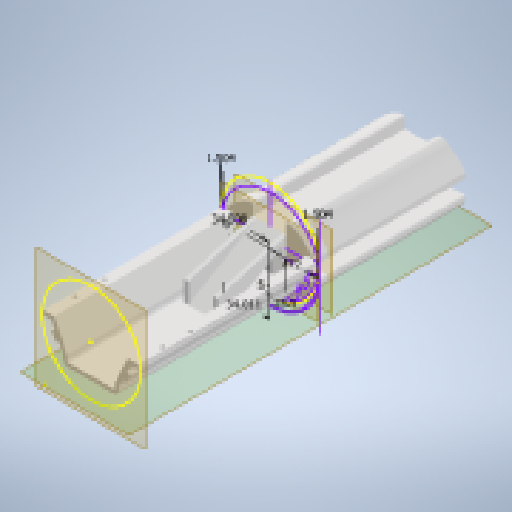
# Autodesk Inventor part: MiddleAdapter_0.5mmOffset
Saved by Autodesk Inventor 2023 (Build 270158030, 158C)
## iProperties
Created: 2022-07-21
Part Number: MiddleAdapter_0.5mmOffset
Material: Generic
Document SubType Name: Modeling
Designer: sqa4002
Density: 1 g/cm^3
Appearance: Default
Author: sqa4002
Autodesk Inventor part; units mm, degrees
ref_plane "YZ Plane" through (0, 0, 0) normal (1, 0, 0) x (0, 1, 0)
ref_plane "XZ Plane" through (0, 0, 0) normal (0, 1, 0) x (-1, 0, 0)
ref_plane "XY Plane" through (0, 0, 0) normal (0, 0, 1) x (1, 0, 0)
sketch "Sketch1" plane through (0, 0, 0) normal (0, 0, 1) x (1, 0, 0)
  arc A0 (19, 57.068098) -> (5, 45.931677) centre (29.5, 29.5) ccw
  arc A1 (63, 45.931677) -> (49, 57.068098) centre (38.5, 29.5) ccw
  line L0 (49, 57.068098) -> (49, 49)
  line L1 (49, 49) -> (19, 49)
  line L2 (19, 49) -> (19, 57.068098)
  line L3 (51, 39.215827) -> (51, 45.931677)
  line L4 (51, 45.931677) -> (63, 45.931677)
  line L5 (5, 45.931677) -> (17, 45.931677)
  line L6 (17, 29) -> (5, 29)
  line L7 (63, 29) -> (51, 29)
  line L8 (51, 29) -> (51, 35.71585)
  line L9 (51, 35.71585) -> (41, 35.71585)
  line L10 (41, 35.71585) -> (41, 39.215827)
  line L11 (41, 39.215827) -> (51, 39.215827)
  line L12 (17, 45.931677) -> (17, 39.215827)
  line L13 (17, 39.215827) -> (27, 39.215827)
  line L14 (27, 39.215827) -> (27, 35.715827)
  line L15 (27, 35.715827) -> (17, 35.715827)
  line L16 (17, 35.715827) -> (17, 29)
  arc A2 (5, 29) -> (63, 29) centre (34, 49.533333) ccw
  point P0 (0, 0)
  point P1 (17, 44.965827)
  point P2 (17, 35.465827)
  point P3 (17, 29.465827)
  point P4 (51, 29.465827)
  point P5 (51, 35.465827)
  point P6 (29.5, 29.5)
  point P7 (38.5, 29.5)
sketch "Sketch7" plane through (0, 0, 0) normal (0, 0, 1) x (1, 0, 0)
  arc A0 (19, 57.068098) -> (5, 45.931677) centre (29.5, 29.5) ccw
  arc A1 (63, 45.931677) -> (49, 57.068098) centre (38.5, 29.5) ccw
  line L0 (49, 57.068098) -> (49, 49)
  line L1 (49, 49) -> (19, 49)
  line L2 (19, 49) -> (19, 57.068098)
  arc A2 (5, 29) -> (63, 29) centre (34, 49.533333) ccw
  line L3 (63, 29) -> (51, 29)
  line L4 (51, 29) -> (51, 35.71585)
  line L5 (51, 29) -> (51, 45.931677)
  line L6 (51, 45.931677) -> (63, 45.931677)
  line L7 (5, 45.931677) -> (17, 45.931677)
  line L8 (17, 45.931677) -> (17, 29)
  line L9 (17, 35.715827) -> (17, 29)
  line L10 (17, 29) -> (5, 29)
  point P0 (0, 0)
  point P1 (0, 0)
  point P2 (38.5, 29.5)
  point P3 (51, 44.965827)
  point P4 (17, 44.965827)
  point P5 (17, 35.465827)
  point P6 (17, 29.465827)
  point P7 (51, 29.465827)
  point P8 (51, 35.465827)
  constraints: 22 end point, 6 point on circle, 3 centre point
sketch "Sketch8" plane through (0, 0, 0) normal (0, 0, 1) x (1, 0, 0)
  line L0 (16.4, 45.331677) -> (16.4, 29.6)
  line L1 (16.4, 29.6) -> (3.862316, 29.6)
  arc A0 (3.862316, 29.6) -> (64.137684, 29.6) centre (34, 49.533333) ccw
  line L2 (64.137684, 29.6) -> (51.6, 29.6)
  line L3 (51.6, 29.6) -> (51.6, 45.331677)
  line L4 (51.6, 45.331677) -> (64.100156, 45.331677)
  arc A1 (64.100156, 45.331677) -> (48.4, 57.925341) centre (38.5, 29.5) ccw
  line L5 (48.4, 57.925341) -> (48.4, 49.6)
  line L6 (48.4, 49.6) -> (19.6, 49.6)
  line L7 (19.6, 49.6) -> (19.6, 57.925341)
  arc A2 (19.6, 57.925341) -> (3.899844, 45.331677) centre (29.5, 29.5) ccw
  line L8 (3.899844, 45.331677) -> (16.4, 45.331677)
  line L9 (13.9, 42.831677) -> (13.9, 32.1)
  line L10 (13.9, 32.1) -> (1.670629, 32.1)
  line L11 (1.670629, 32.1) -> (1.670629, 28.382773)
  arc A3 (1.670629, 28.382773) -> (66.329371, 28.382773) centre (34, 49.533333) ccw
  line L12 (66.329371, 28.382773) -> (66.329371, 32.1)
  line L13 (66.329371, 32.1) -> (54.1, 32.1)
  line L14 (54.1, 32.1) -> (54.1, 42.831677)
  line L15 (54.1, 42.831677) -> (66.314291, 42.831677)
  line L16 (66.314291, 42.831677) -> (66.314291, 46.503682)
  arc A4 (66.314291, 46.503682) -> (49.244541, 60.27848) centre (38.5, 29.5) ccw
  line L17 (49.244541, 60.27848) -> (45.9, 60.27848)
  line L18 (45.9, 60.27848) -> (45.9, 52.1)
  line L19 (45.9, 52.1) -> (22.1, 52.1)
  line L20 (22.1, 52.1) -> (22.1, 60.27848)
  line L21 (22.1, 60.27848) -> (18.755459, 60.27848)
  arc A5 (18.755459, 60.27848) -> (1.685709, 46.503682) centre (29.5, 29.5) ccw
  line L22 (1.685709, 46.503682) -> (1.685709, 42.831677)
  line L23 (1.685709, 42.831677) -> (13.9, 42.831677)
  point P0 (0, 0)
  point P1 (38.5, 29.5)
  constraints: 48 end point, 12 point on circle, 6 centre point, 6 perpendicular
extrude "Extrusion3" add sketch "Sketch8" along normal blind 100
ref_plane "Work Plane3" through (0, 0, 100) normal (0, 0, 1) x (1, 0, 0)
sketch "Sketch10" plane through (0, 0, 100) normal (0, 0, 1) x (1, 0, 0)
  line L0 (2.035709, 46.404887) -> (2.035709, 43.181677)
  line L1 (2.035709, 43.181677) -> (14.25, 43.181677)
  line L2 (14.25, 43.181677) -> (14.25, 31.75)
  line L3 (14.25, 31.75) -> (2.020629, 31.75)
  line L4 (2.020629, 31.75) -> (2.020629, 28.48735)
  arc A0 (2.020629, 28.48735) -> (65.979371, 28.48735) centre (34, 49.533333) ccw
  line L5 (65.979371, 28.48735) -> (65.979371, 31.75)
  line L6 (65.979371, 31.75) -> (53.75, 31.75)
  line L7 (53.75, 31.75) -> (53.75, 43.181677)
  line L8 (53.75, 43.181677) -> (65.964291, 43.181677)
  line L9 (65.964291, 43.181677) -> (65.964291, 46.404887)
  arc A1 (65.964291, 46.404887) -> (49.185041, 59.92848) centre (38.5, 29.5) ccw
  line L10 (49.185041, 59.92848) -> (46.25, 59.92848)
  line L11 (46.25, 59.92848) -> (46.25, 51.75)
  line L12 (46.25, 51.75) -> (21.75, 51.75)
  line L13 (21.75, 51.75) -> (21.75, 59.92848)
  line L14 (21.75, 59.92848) -> (18.814959, 59.92848)
  arc A2 (18.814959, 59.92848) -> (2.035709, 46.404887) centre (29.5, 29.5) ccw
  line L15 (4.520629, 29.25) -> (16.75, 29.25)
  line L16 (16.75, 29.25) -> (16.75, 45.681677)
  line L17 (16.75, 45.681677) -> (4.535709, 45.681677)
  arc A3 (19.25, 57.42848) -> (4.535709, 45.681677) centre (29.5, 29.5) ccw
  line L18 (19.25, 57.42848) -> (19.25, 49.25)
  line L19 (19.25, 49.25) -> (48.75, 49.25)
  line L20 (48.75, 49.25) -> (48.75, 57.42848)
  arc A4 (63.464291, 45.681677) -> (48.75, 57.42848) centre (38.5, 29.5) ccw
  line L21 (63.464291, 45.681677) -> (51.25, 45.681677)
  line L22 (51.25, 45.681677) -> (51.25, 29.25)
  line L23 (51.25, 29.25) -> (63.479371, 29.25)
  arc A5 (4.520629, 29.25) -> (63.479371, 29.25) centre (34, 49.533333) ccw
  line L24 (13.9, 32.1) -> (1.670629, 32.1)
  line L25 (1.670629, 32.1) -> (1.670629, 28.382773)
  arc A6 (1.670629, 28.382773) -> (66.329371, 28.382773) centre (34, 49.533333) ccw
  line L26 (66.329371, 28.382773) -> (66.329371, 32.1)
  line L27 (66.329371, 32.1) -> (54.1, 32.1)
  line L28 (54.1, 32.1) -> (54.1, 42.831677)
  line L29 (54.1, 42.831677) -> (66.314291, 42.831677)
  line L30 (66.314291, 42.831677) -> (66.314291, 46.503682)
  arc A7 (66.314291, 46.503682) -> (49.244541, 60.27848) centre (38.5, 29.5) ccw
  line L31 (49.244541, 60.27848) -> (45.9, 60.27848)
  line L32 (45.9, 60.27848) -> (45.9, 52.1)
  line L33 (45.9, 52.1) -> (22.1, 52.1)
  line L34 (22.1, 52.1) -> (22.1, 60.27848)
  line L35 (22.1, 60.27848) -> (18.755459, 60.27848)
  arc A8 (18.755459, 60.27848) -> (1.685709, 46.503682) centre (29.5, 29.5) ccw
  line L36 (1.685709, 46.503682) -> (1.685709, 42.831677)
  line L37 (1.685709, 42.831677) -> (13.9, 42.831677)
  line L38 (13.9, 42.831677) -> (13.9, 32.1)
  line L39 (16.4, 45.331677) -> (3.899844, 45.331677)
  arc A9 (19.6, 57.925341) -> (3.899844, 45.331677) centre (29.5, 29.5) ccw
  line L40 (19.6, 57.925341) -> (19.6, 49.6)
  line L41 (19.6, 49.6) -> (48.4, 49.6)
  line L42 (48.4, 49.6) -> (48.4, 57.925341)
  arc A10 (64.100156, 45.331677) -> (48.4, 57.925341) centre (38.5, 29.5) ccw
  line L43 (64.100156, 45.331677) -> (51.6, 45.331677)
  line L44 (51.6, 45.331677) -> (51.6, 29.6)
  line L45 (51.6, 29.6) -> (64.137684, 29.6)
  arc A11 (3.862316, 29.6) -> (64.137684, 29.6) centre (34, 49.533333) ccw
  line L46 (3.862316, 29.6) -> (16.4, 29.6)
  line L47 (16.4, 29.6) -> (16.4, 45.331677)
  point P0 (0, 0)
extrude "Extrusion4" add sketch "Sketch10" along normal blind 10 contours A2 L14 L13 L12 L11 L10 A1 L9 L8 L7 L6 L5 A0 L4 L3 L2 L1 L0 | L15 L16 L17 A3 L18 L19 L20 A4 L21 L22 L23 A5 | L38 L37 L36 A8 L35 L34 L33 L32 L31 A7 L30 L29 L28 L27 L26 A6 L25 L24 | L39 A9 L40 L41 L42 A10 L43 L44 L45 A11 L46 L47
sketch "Sketch11" plane through (0, 0, 110) normal (0, 0, 1) x (1, 0, 0)
  line L0 (5.317303, 37.465838) -> (7.794293, 32.202234)
  line L1 (7.794293, 32.202234) -> (5.351283, 31.052582)
  line L2 (5.351283, 31.052582) -> (8.331862, 24.718851)
  line L3 (8.331862, 24.718851) -> (10.774872, 25.868503)
  line L4 (10.774872, 25.868503) -> (13.5, 20.077607)
  line L5 (13.5, 20.077607) -> (13.5, 17.965838)
  arc A0 (13.5, 17.965838) -> (18, 13.465838) centre (18, 17.965838) ccw
  line L6 (18, 13.465838) -> (50, 13.465838)
  arc A1 (50, 13.465838) -> (54.5, 17.965838) centre (50, 17.965838) ccw
  line L7 (54.5, 17.965838) -> (54.5, 20.077607)
  line L8 (54.5, 20.077607) -> (57.225128, 25.868503)
  line L9 (57.225128, 25.868503) -> (59.668138, 24.718851)
  line L10 (59.668138, 24.718851) -> (62.648717, 31.052582)
  line L11 (62.648717, 31.052582) -> (60.205707, 32.202234)
  line L12 (60.205707, 32.202234) -> (62.682697, 37.465838)
  line L13 (62.682697, 37.465838) -> (68.496377, 37.465838)
  arc A2 (-0.496377, 37.465838) -> (68.496377, 37.465838) centre (34, 36.965838) ccw
  line L14 (-0.496377, 37.465838) -> (5.317303, 37.465838)
  circle A3 centre (34, 8.465838) radius 2.75
  circle A4 centre (34.011144, 37.465838) radius 36
  line L15 (34.011144, 1.465838) -> (34.011144, 73.465838)
  line L16 (70.011144, 37.465838) -> (-1.988856, 37.465838)
  line L17 (69.999977, 73.499564) -> (69.999977, 1.499564)
  line L18 (-1.999977, 1.499564) -> (-1.999977, 73.499564)
  point P0 (0, 0)
  point P1 (-1.48044, 45.569992)
  point P2 (34, 13.465838)
  point P3 (69.48044, 45.569992)
  point P4 (-0.443994, 38.930856)
  point P5 (68.443994, 38.930856)
  point P6 (0.816224, 46.40443)
  point P7 (67.183776, 46.40443)
  point P8 (0, 0)
  dimension "d27" = 5
  dimension "d28" = 28.5
  dimension "d31" = 72
  dimension "d35" = 1.5036
  dimension "d36" = 1.5036
  dimension "d37" = 34.50752
  dimension "d38" = 0
  dimension "d39" = 34.01114
  constraints: 38 end point, 14 point on circle, 5 centre point, 2 perpendicular, 2 point on line, 2 vertical, 1 midpoint
  measures "d27" distance of point (34, 13.466) A3.centre
  measures "d28" distance of A2.centre A3.centre
  measures "d31" diameter of A4
  measures "d35" distance from line of L18 L14.start
  measures "d36" distance from line of L17 L13.end
  measures "d37" distance of A4.centre L14.start
  measures "d38" distance between parallel lines of L16 L14
  measures "d39" horizontal distance of point (0, 0) A4.centre
sketch "Sketch12" plane through (0, 0, 110) normal (0, 0, 1) x (1, 0, 0)
  circle A0 centre (34, 43.5) radius 36
  line L0 (34, 79.5) -> (34, 7.5)
  line L1 (70, 43.5) -> (-2, 43.5)
  arc A1 (-0.496377, 43.5) -> (68.496377, 43.5) centre (34, 43) ccw
  line L2 (5.317303, 43.5) -> (7.794293, 38.236396)
  line L3 (7.794293, 38.236396) -> (5.351283, 37.086744)
  line L4 (5.351283, 37.086744) -> (8.331862, 30.753013)
  line L5 (8.331862, 30.753013) -> (10.774872, 31.902665)
  line L6 (10.774872, 31.902665) -> (13.5, 26.111768)
  line L7 (13.5, 26.111768) -> (13.5, 24)
  arc A2 (13.5, 24) -> (18, 19.5) centre (18, 24) ccw
  line L8 (18, 19.5) -> (50, 19.5)
  arc A3 (50, 19.5) -> (54.5, 24) centre (50, 24) ccw
  line L9 (54.5, 24) -> (54.5, 26.111768)
  line L10 (54.5, 26.111768) -> (57.225128, 31.902665)
  line L11 (57.225128, 31.902665) -> (59.668138, 30.753013)
  line L12 (59.668138, 30.753013) -> (62.648717, 37.086744)
  line L13 (62.648717, 37.086744) -> (60.205707, 38.236396)
  line L14 (60.205707, 38.236396) -> (62.682697, 43.5)
  line L15 (62.682697, 43.5) -> (68.496377, 43.5)
  circle A4 centre (34, 14.5) radius 2.75
  line L16 (5.317303, 43.5) -> (-0.496377, 43.5)
  point P0 (0, 0)
  point P1 (-0.250325, 38.856906)
  point P2 (68.250325, 38.856906)
  point P3 (-0.329941, 46.421278)
  point P4 (68.329941, 46.421278)
  point P5 (0.881853, 46.584282)
  point P6 (34, 19.5)
  point P7 (67.118147, 46.584282)
  dimension "d42" = 5
  dimension "d43" = 28.5
  dimension "d44" = 0
  constraints: 34 end point, 14 point on circle, 4 centre point, 2 point on line, 1 horizontal, 1 midpoint, 1 vertical
  measures "d42" distance of point (34, 19.5) A4.centre
  measures "d43" distance of A1.centre A4.centre
  measures "d44" distance between parallel lines of L1 L16
ref_plane "Work Plane4" through (0, 0, 110) normal (0, 0, 1) x (1, 0, 0)
sketch "Sketch13" plane through (0, 0, 110) normal (0, 0, 1) x (1, 0, 0)
  circle A0 centre (34, 43.5) radius 36
  line L0 (34, 79.5) -> (34, 7.5)
  line L1 (70, 43.5) -> (-2, 43.5)
  line L2 (5.467102, 43.181677) -> (14.25, 43.181677)
  line L3 (5.317303, 43.5) -> (7.794293, 38.236396)
  arc A1 (-0.496377, 43.5) -> (68.496377, 43.5) centre (34, 43) ccw
  line L4 (7.794293, 38.236396) -> (5.351283, 37.086744)
  line L5 (5.351283, 37.086744) -> (8.331862, 30.753013)
  line L6 (8.331862, 30.753013) -> (10.774872, 31.902665)
  line L7 (10.774872, 31.902665) -> (13.5, 26.111768)
  line L8 (13.5, 26.111768) -> (13.5, 24)
  arc A2 (13.5, 24) -> (18, 19.5) centre (18, 24) ccw
  line L9 (18, 19.5) -> (50, 19.5)
  circle A3 centre (34, 14.5) radius 2.75
  arc A4 (50, 19.5) -> (54.5, 24) centre (50, 24) ccw
  line L10 (54.5, 24) -> (54.5, 26.111768)
  line L11 (54.5, 26.111768) -> (57.225128, 31.902665)
  line L12 (57.225128, 31.902665) -> (59.668138, 30.753013)
  line L13 (59.668138, 30.753013) -> (62.648717, 37.086744)
  line L14 (62.648717, 37.086744) -> (60.205707, 38.236396)
  line L15 (60.205707, 38.236396) -> (62.682697, 43.5)
  line L16 (62.682697, 43.5) -> (68.496377, 43.5)
  line L17 (5.317303, 43.5) -> (-0.496377, 43.5)
  line L18 (5.467102, 43.181677) -> (14.25, 43.181677)
  line L19 (14.25, 43.181677) -> (14.25, 31.75)
  line L20 (14.25, 31.75) -> (2.020629, 31.75)
  line L21 (2.020629, 31.75) -> (2.020629, 28.48735)
  arc A5 (2.020629, 28.48735) -> (65.979371, 28.48735) centre (34, 49.533333) ccw
  line L22 (65.979371, 28.48735) -> (65.979371, 31.75)
  line L23 (65.979371, 31.75) -> (53.75, 31.75)
  line L24 (53.75, 31.75) -> (53.75, 43.181677)
  line L25 (53.75, 43.181677) -> (62.532898, 43.181677)
  line L26 (49.185041, 59.92848) -> (46.25, 59.92848)
  line L27 (46.25, 59.92848) -> (46.25, 51.75)
  line L28 (46.25, 51.75) -> (21.75, 51.75)
  line L29 (21.75, 51.75) -> (21.75, 59.92848)
  line L30 (21.75, 59.92848) -> (18.814959, 59.92848)
  line L31 (12.211937, 35.894512) -> (7.181457, 46.584282)
  line L32 (60.77832, 46.584282) -> (55.788063, 35.894512)
  line L33 (55.788063, 35.894512) -> (51.5, 26.782379)
  line L34 (51.5, 26.782379) -> (51.5, 24)
  arc A6 (50, 22.5) -> (51.5, 24) centre (50, 24) ccw
  line L35 (50, 22.5) -> (18, 22.5)
  arc A7 (16.5, 24) -> (18, 22.5) centre (18, 24) ccw
  line L36 (16.5, 24) -> (16.5, 26.782379)
  line L37 (16.5, 26.782379) -> (12.211937, 35.894512)
  arc A8 (67.118147, 46.584282) -> (49.185041, 59.92848) centre (44.1845, 34.486172) ccw
  arc A9 (18.814959, 59.92848) -> (0.881853, 46.584282) centre (23.8155, 34.486172) ccw
  line L38 (7.181457, 46.584282) -> (0.881853, 46.584282)
  line L39 (60.77832, 46.584282) -> (67.118147, 46.584282)
  line L40 (-0.496377, 43.5) -> (-0.496377, 46.584282)
  line L41 (-0.496377, 46.584282) -> (0.881853, 46.584282)
  line L42 (68.496377, 43.5) -> (68.496377, 46.584282)
  line L43 (68.496377, 46.584282) -> (67.118147, 46.584282)
  point P0 (0, 0)
  point P1 (0, 0)
  point P2 (-0.250325, 38.856906)
  point P3 (68.250325, 38.856906)
  point P4 (-0.329941, 46.421278)
  point P5 (68.329941, 46.421278)
  point P6 (34, 19.5)
  point P7 (-0.496377, 43.5)
  point P8 (68.496377, 43.5)
  dimension "d46" = 5
  dimension "d47" = 28.5
  dimension "d48" = 0
  constraints: 88 end point, 24 point on circle, 10 centre point, 4 point on line, 2 collinear, 2 perpendicular, 2 vertical, 1 horizontal, 1 midpoint, 1 parallel, 6 other
  measures "d46" distance of point (34, 19.5) A3.centre
  measures "d47" distance of A1.centre A3.centre
  measures "d48" distance between parallel lines of L1 L17
extrude "Extrusion5" add sketch "Sketch13" along normal blind 130 contours L1 L32 L39 L43 L42 | L15 L25 L32 L1 | L40 L41 L38 L31 L1 | L15 L14 L13 L23 L12 L11 L33 L32 L25 | L1 L31 L2 L3 | L35 A6 L34 L33 L23 L11 L10 A4 L9 L0 | L0 L9 A2 L8 L7 L20 L37 L36 A7 L35 | L13 L12 L23 | L2 L31 L37 L20 L7 L6 L5 L4 L3 | L20 L6 L5
sketch "Sketch14" plane through (18, 22.5, 110) normal (0, 1, 0) x (1, 0, 0)
  line L0 (28.25, 0) -> (3.75, 0) projected
  line L1 (3.75, 0) -> (28.25, 0)
  line L2 (0, 0) -> (32, 0) projected
  line L3 (28.25, 0) -> (28.25, -50)
  line L4 (32, 0) -> (32, -130) projected
  line L5 (32, -130) -> (0, -130) projected
  line L6 (3.75, 0) -> (3.75, -50)
  line L7 (32, 0) -> (0, 0) projected
  line L8 (25.25, -50) -> (25.25, 0)
  line L9 (6.75, 0) -> (6.75, -50)
  line L10 (28.25, -50) -> (25.25, -50)
  line L11 (6.75, -50) -> (3.75, -50)
  point P0 (-18, 110)
  dimension "d62" = 3
  dimension "d121" = 50
  constraints: 14 end point, 6 point on line, 2 perpendicular, 1 collinear, 1 parallel
  measures "d62" distance between parallel lines of L6 L9
  measures "d121" distance between parallel lines of L0 L10
ref_plane "Work Plane5" through (24.75, 22.5, 110) normal (0, 1, 0) x (1, 0, 0)
sketch "Sketch15" plane through (24.75, 22.5, 110) normal (0, 1, 0) x (1, 0, 0)
  line L0 (0, 0) -> (18.5, 0) projected
  line L1 (18.5, 0) -> (18.5, -130) projected
  line L2 (0, 0) -> (18.5, 0)
  line L3 (18.5, 0) -> (18.5, -50)
  line L4 (0, 0) -> (0, -130) projected
  line L5 (0, -50) -> (0, 0)
  line L6 (18.5, -50) -> (0, -50)
  point P0 (-24.75, 110)
  point P1 (0, -50)
  point P2 (18.5, -50)
  dimension "d120" = 50
  constraints: 8 end point, 3 perpendicular, 1 collinear
  measures "d120" distance between parallel lines of L6 L0
fillet "Fillet2" radius 1 19 edges at (22.1, 60.2785, 55) (18.7555, 60.2785, 55) (45.9, 60.2785, 55) (49.2445, 60.2785, 55) (1.6857, 46.5037, 55) (1.6857, 42.8317, 55) (1.6706, 32.1, 55) (1.6706, 28.3828, 55) (34, 10.9, 110) (4.6843, 32.1, 110) (1.6706, 30.2414, 110) (66.3294, 30.2414, 110) (63.3157, 32.1, 110) (66.3294, 32.1, 55) (66.3294, 28.3828, 55) (58.9359, 54.8995, 110) (9.0641, 54.8995, 110) (20.4277, 60.2785, 110) (47.5723, 60.2785, 110)
ref_plane "Work Plane6" through (13.9, 32.1, 0) normal (-1, 0, 0) x (0, 0, 1)
sketch "Sketch17" plane through (13.9, 32.1, 0) normal (-1, 0, 0) x (0, 0, 1)
  circle A0 centre (20, 5.365838) radius 3
  circle A1 centre (40, 5.365838) radius 3
  line L0 (0, 10.731677) -> (0, 0)
  point P0 (0, -32.1)
  dimension "d98" = 6
  dimension "d99" = 6
  dimension "d100" = 20
  dimension "d101" = 20
  constraints: 2 centre point
  measures "d98" diameter of A0
  measures "d99" diameter of A1
  measures "d100" distance from line of L0 A0.centre
  measures "d101" distance of A0.centre A1.centre
extrude "Extrusion11" cut sketch "Sketch17" against normal through all
ref_plane "Work Plane7" through (34, 10.9, 0) normal (0, -1, 0) x (1, 0, 0)
sketch "Sketch18" plane through (34, 10.9, 0) normal (0, -1, 0) x (1, 0, 0)
  circle A0 centre (0, 20) radius 4
  line L0 (32.161861, 0) -> (-32.161861, 0)
  circle A1 centre (0, 40) radius 4
  point P0 (-34, 0)
  dimension "d104" = 8
  dimension "d105" = 20
  dimension "d106" = 8
  dimension "d107" = 20
  constraints: 2 centre point
  measures "d104" diameter of A0
  measures "d105" distance from line of L0 A0.centre
  measures "d106" diameter of A1
  measures "d107" distance of A0.centre A1.centre
extrude "Extrusion12" cut sketch "Sketch18" against normal blind 3
ref_plane "Work Plane8" through (34, 33.042141, 240) normal (0, 0, 1) x (1, 0, 0)
sketch "Sketch19" plane through (34, 33.042141, 240) normal (0, 0, 1) x (1, 0, 0)
  point P0 (-34, -33.042141)
sketch "Sketch20" plane through (34, 33.042141, 240) normal (0, 0, 1) x (1, 0, 0)
  circle A0 centre (0, 10.457859) radius 36
  point P0 (-34, -33.042141)
sketch "Sketch21" plane through (60.77832, 46.584282, 240) normal (0, 1, 0) x (1, 0, 0)
  circle A0 centre (5.218056, 20) radius 1.5
  circle A1 centre (5.218056, 40) radius 1.5
  circle A2 centre (-58.774697, 20) radius 1.5
  circle A3 centre (-58.774697, 41.5) radius 1.5
  line L0 (7.718056, 0) -> (0, 0)
  line L1 (-53.596863, 0) -> (-61.274697, 0)
  line L2 (-61.274697, 130) -> (-61.274697, 0)
  line L3 (7.718056, 130) -> (7.718056, 0)
  point P0 (-60.77832, 240)
  dimension "d110" = 3
  dimension "d111" = 3
  dimension "d112" = 3
  dimension "d113" = 3
  dimension "d114" = 20
  dimension "d115" = 40
  dimension "d116" = 20
  dimension "d117" = 40
  dimension "d123" = 2.5
  dimension "d124" = 2.5
  dimension "d125" = 2.5
  dimension "d126" = 2.5
  constraints: 4 centre point
  measures "d110" diameter of A0
  measures "d111" diameter of A1
  measures "d112" diameter of A2
  measures "d113" diameter of A3
  measures "d114" distance from line of A0.centre L0
  measures "d115" distance from line of A1.centre L0
  measures "d116" distance from line of A2.centre L1
  measures "d117" distance edge to line of A3 L1
  measures "d123" distance from line of L2 A2.centre
  measures "d124" distance from line of L2 A3.centre
  measures "d125" distance from line of L3 A0.centre
  measures "d126" distance from line of L3 A1.centre
extrude "Extrusion13" cut sketch "Sketch21" against normal through all
extrude "Extrusion15" add sketch "Sketch15" along normal blind 29.6
chamfer "Chamfer11" distance 50 distance2 29.6 1 edges at (34, 52.1, 160) measured on face at (34, 52.1, 159.5)
extrude "Extrusion16" add sketch "Sketch14" along normal blind 29.6
chamfer "Chamfer12" distance 50 distance2 14.8 2 edges at (44.75, 52.1, 160) (23.25, 52.1, 160) measured on face at (23.25, 52.1, 159.5) measured on face at (44.75, 52.1, 159.5)
sketch "Sketch23" plane through (21.75, 22.5, 110) normal (-1, 0, 0) x (0, 0, 1)
  line L0 (0, 29.6) -> (0, 29.6)
  line L1 (50, 0) -> (0, 0)
  line L2 (0, 29.6) -> (0, 0)
  line L3 (0, 0) -> (50, 0)
  line L4 (50, 0) -> (0, 29.6)
  line L5 (5, 5) -> (5, 20.829527)
  line L6 (5, 20.829527) -> (31.739065, 5)
  line L7 (31.739065, 5) -> (5, 5)
  point P0 (-110, -22.5)
  dimension "d149" = 5
  constraints: 12 end point, 2 perpendicular, 1 vertical, 2 other
  measures "d149" distance between parallel lines of L2 L5
extrude "Extrusion17" cut sketch "Sketch23" against normal up to surface (24.5 mm away) contours L5 L6 L7
chamfer "Chamfer13" distance 2 distance2 5 3 edges at (21.75, 35.4148, 115) (21.75, 35.4148, 128.3695) (21.75, 27.5, 128.3695) measured on face at (21.75, 35.4148, 114.5) measured on face at (21.75, 35.845, 128.6242) measured on face at (21.75, 27, 128.3695)
chamfer "Chamfer14" distance 2 distance2 5 3 edges at (46.25, 35.4148, 115) (46.25, 27.5, 128.3695) (46.25, 35.4148, 128.3695) measured on face at (46.25, 35.4148, 114.5) measured on face at (46.25, 35.845, 128.6242) measured on face at (46.25, 27, 128.3695)
body "Solid2"
